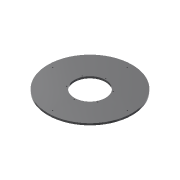
# Autodesk Inventor part: Диск_опорный
Saved by Autodesk Inventor 2022 (Build 260153000, 153)
## iProperties
RuleStatus: InUse
Part Number: Диск_опорный
Checked By: Якушев
Engr Approved By: Малов
Material: По умолчанию1
Document SubType Name: Modeling
Mfg Approved By: Судаков
Designer: Смирнов
Density: 1 g/cm^3
Appearance: Гладкий — нейтральный серый
AfterMaterialChange0: Материал
BeforeDocSave0: Материал
AfterAnyiPropertyChange0: Материал
Материал: По умолчанию1
Author: Смирнов
Autodesk Inventor part; units mm, degrees
ref_plane "YZ Plane" through (0, 0, 0) normal (1, 0, 0) x (0, 1, 0)
ref_plane "XZ Plane" through (0, 0, 0) normal (0, 1, 0) x (-1, 0, 0)
ref_plane "XY Plane" through (0, 0, 0) normal (0, 0, 1) x (1, 0, 0)
sketch "Эскиз1" plane through (0, 0, 0) normal (0, 0, 1) x (1, 0, 0)
  circle A0 centre (0, 0) radius 135
  dimension "d0" = 270
  constraints: 1 centre point, 1 coincident
  measures "d0" diameter of A0
extrude "Выдавливание1" add sketch "Эскиз1" along normal mid plane 6
sketch "Эскиз2" plane through (0, 0, 3) normal (0, 0, 1) x (1, 0, 0)
  circle A0 centre (0, 0) radius 120 construction
  line L0 (0, 0) -> (0, -223.6058) construction
  point P0 (0, -120)
  dimension "d3" = 240
  constraints: 2 end point, 1 coincident, 1 point on line, 1 vertical, 1 vertical alignment, 2 other
hole "Отверстие1" at (0, -120, 3) direction (0, 0, -1) diameter 3.2 end through all clearance for "лты с шестигранной головкой / гайка ГОСТ 12876-67" size "M3" standard "ГОСТ"
pattern_circular "Круговой массив1" count 4 over 360 about axis through (0, 0, 0) along (0, 0, 1) of "Отверстие1"
sketch "Эскиз3" plane through (0, 0, -3) normal (0, 0, -1) x (-1, 0, 0)
  circle A0 centre (0, 0) radius 50
  dimension "d14" = 100
  constraints: 1 centre point, 1 coincident
  measures "d14" diameter of A0
extrude "Выдавливание2" cut sketch "Эскиз3" against normal through all
sketch "Эскиз4" plane through (0, 0, -3) normal (0, 0, -1) x (-1, 0, 0)
  circle A0 centre (44.8931, -30.0102) radius 2.25 construction
  point P0 (0, 0)
hole "Отверстие2" at (-44.8931, -30.0102, -3) direction (0, 0, 1) diameter 3.4 end through all
pattern_circular "Круговой массив2" count 6 over 360 about axis through (0, 0, -3) along (0, 0, 1) of "Отверстие2"
